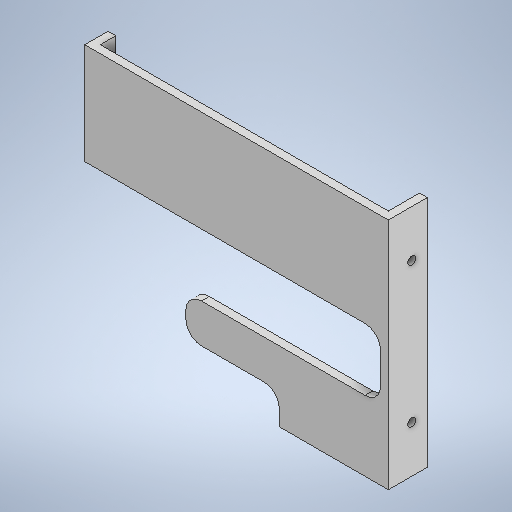
# Autodesk Inventor part: tright
Saved by Autodesk Inventor 2026.1 (Build 301233000, 233)
## iProperties
Created: 2026-05-31
Part Number: tright
Material: Generic
Document SubType Name: Modeling
Designer: chris
Density: 1 g/cm^3
Appearance: Default
Author: chris
Autodesk Inventor part; units mm, degrees
ref_plane "YZ Plane" through (0, 0, 0) normal (1, 0, 0) x (0, 1, 0)
ref_plane "XZ Plane" through (0, 0, 0) normal (0, 1, 0) x (-1, 0, 0)
ref_plane "XY Plane" through (0, 0, 0) normal (0, 0, 1) x (1, 0, 0)
sketch "Sketch1" plane through (0, 0, 0) normal (0, 0, 1) x (1, 0, 0)
  line L0 (-97.5, -75) -> (97.5, -75)
  line L1 (97.5, -75) -> (97.5, 75)
  line L2 (97.5, 75) -> (-97.5, 75)
  line L3 (-97.5, 75) -> (-97.5, -75)
  line L4 (-97.5, -75) -> (-32.5, -30) construction
  line L5 (97.5, -75) -> (-97.5, 75) construction
  line L6 (-97.5, -75) -> (-32.5, -75)
  line L7 (-32.5, -45) -> (-32.5, -40)
  line L8 (-42.5, 10) -> (-97.5, 10)
  line L9 (-97.5, 10) -> (-97.5, -75)
  line L10 (-97.5, -75) -> (27.5, -75)
  line L11 (27.5, -75) -> (27.5, -65)
  line L12 (17.5, -55) -> (-22.5, -55)
  line L13 (-97.5, -55) -> (-97.5, -75)
  arc A0 (-32.5, -45) -> (-22.5, -55) centre (-22.5, -45) ccw
  arc A1 (27.5, -65) -> (17.5, -55) centre (17.5, -65) ccw
  line L14 (-42.5, 10) -> (82.5, 10)
  line L15 (92.5, 0) -> (92.5, -20)
  line L16 (82.5, -30) -> (-22.5, -30)
  line L17 (-32.5, -30) -> (97.5, 75) construction
  arc A2 (-22.5, -30) -> (-32.5, -40) centre (-22.5, -40) ccw
  arc A3 (82.5, -30) -> (92.5, -20) centre (82.5, -20) ccw
  arc A4 (92.5, 0) -> (82.5, 10) centre (82.5, 0) ccw
  point P0 (0, 0)
  point P1 (-32.5, 10)
  point P2 (27.5, -55)
  point P3 (92.5, -30)
  point P4 (92.5, 10)
  dimension "d0" = 195
  dimension "d1" = 150
  dimension "d2" = 65
  dimension "d3" = 85
  dimension "d4" = 125
  dimension "d5" = 20
  dimension "d36" = 40
  dimension "d37" = 190
  dimension "d38" = 10
  constraints: 36 end point, 12 point on line, 10 point on circle, 10 tangent, 7 parallel, 5 centre point, 4 horizontal, 4 perpendicular, 3 equal radius, 1 midpoint
  measures "d0" distance of L2.end L1.end
  measures "d1" distance of L0.end L1.end
  measures "d2" distance of L8.end point (-32.5, 10)
  measures "d3" distance of point (-32.5, 10) L6.end
  measures "d4" distance of L13.start point (27.5, -55)
  measures "d5" distance of point (27.5, -55) L10.end
  measures "d36" distance of point (92.5, 10) point (92.5, -30)
  measures "d37" distance between parallel lines of L15 L9
  measures "d38" radius of A2
extrude "Extrusion1" add sketch "Sketch1" along normal blind 5 contours L11 A1 L12 A0 L7 A2 L16 A3 L15 A4 L14 L8 L3 L2 L1 L0
sketch "Sketch2" plane through (0, 0, 0) normal (0, 0, -1) x (-1, 0, 0)
  line L0 (92.5, 75) -> (97.5, 75)
  line L1 (97.5, 75) -> (97.5, 10)
  line L2 (97.5, 10) -> (92.5, 10)
  line L3 (92.5, 10) -> (92.5, 75)
  line L4 (-97.5, 75) -> (97.5, 75) projected
  line L5 (97.5, 10) -> (-82.5, 10) projected
  line L6 (97.5, 75) -> (97.5, 10) projected
  point P0 (0, 0)
  point P1 (42.5, 5)
  point P2 (97.5, -75)
  point P3 (-82.5, 10)
  dimension "d9" = 5
  constraints: 8 end point, 2 collinear, 2 horizontal, 2 parallel, 1 perpendicular, 1 other
  measures "d9" distance of L1.end L2.end
extrude "Extrusion2" add sketch "Sketch2" along normal blind 10
sketch "Sketch3" plane through (0, 0, 0) normal (0, 0, -1) x (-1, 0, 0)
  line L0 (-97.5, 75) -> (-92.5, 75)
  line L1 (-92.5, 75) -> (-92.5, -75)
  line L2 (-92.5, -75) -> (-97.5, -75)
  line L3 (-97.5, -75) -> (-97.5, 75)
  line L4 (-97.5, -70) -> (-27.5, -70)
  line L5 (-27.5, -70) -> (-27.5, -75)
  line L6 (-27.5, -75) -> (-97.5, -75)
  line L7 (-97.5, -75) -> (-97.5, -70)
  line L8 (-97.5, -75) -> (-97.5, 75) projected
  line L9 (-97.5, 75) -> (92.5, 75) projected
  line L10 (-27.5, -75) -> (-97.5, -75) projected
  line L11 (-27.5, -65) -> (-27.5, -75) projected
  point P0 (0, 0)
  point P1 (-92.5, -70)
  point P2 (97.5, -75)
  dimension "d12" = 5
  dimension "d13" = 5
  constraints: 16 end point, 5 collinear, 4 parallel, 2 horizontal, 2 perpendicular, 1 point on line
  measures "d12" distance of L0.start L0.end
  measures "d13" distance of L4.end L5.end
extrude "Extrusion3" add sketch "Sketch3" along normal blind 20
sketch "Sketch4" plane through (97.5, -75, 5) normal (1, 0, 0) x (0, 0, -1)
  circle A0 centre (15, 30) radius 2.55
  circle A1 centre (15, 120) radius 2.55
  line L0 (0, 0) -> (0, 150) projected
  line L1 (25, 0) -> (0, 0) projected
  point P0 (5, 75)
  dimension "d16" = 5.1
  dimension "d17" = 5.1
  dimension "d18" = 15
  dimension "d19" = 30
  dimension "d20" = 90
  constraints: 2 centre point, 1 vertical alignment
  measures "d16" diameter of A0
  measures "d17" diameter of A1
  measures "d18" distance from line of L0 A0.centre
  measures "d19" distance from line of L1 A0.centre
  measures "d20" distance of A0.centre A1.centre
extrude "Extrusion4" cut sketch "Sketch4" against normal blind 20
sketch "Sketch5" plane through (27.5, -75, 5) normal (0, -1, 0) x (1, 0, 0)
  circle A0 centre (35, -15) radius 2.55
  line L0 (70, -25) -> (70, 0) projected
  line L1 (0, 0) -> (70, 0) projected
  point P0 (-27.5, -5)
  point P1 (70, -12.5)
  point P2 (35, 0)
  point P3 (-125, 0)
  dimension "d23" = 5.1
  dimension "d24" = 35
  dimension "d25" = 15
  constraints: 2 midpoint, 1 centre point
  measures "d23" diameter of A0
  measures "d24" horizontal distance of point (70, -12.5) A0.centre
  measures "d25" distance of point (35, 0) A0.centre
extrude "Extrusion5" cut sketch "Sketch5" against normal blind 20
sketch "Sketch6" plane through (-97.5, 10, 5) normal (-1, 0, 0) x (0, 0, 1)
  circle A0 centre (-10, 45) radius 2.05
  circle A1 centre (-10, 20) radius 2.05
  line L0 (-15, 0) -> (-15, 65) projected
  line L1 (-15, 0) -> (0, 0) projected
  line L2 (0, 65) -> (-15, 65) projected
  point P0 (-5, -10)
  dimension "d28" = 4.1
  dimension "d29" = 4.1
  dimension "d30" = 5
  dimension "d31" = 20
  dimension "d32" = 20
  constraints: 2 centre point, 1 vertical alignment
  measures "d28" diameter of A0
  measures "d29" diameter of A1
  measures "d30" distance from line of L0 A1.centre
  measures "d31" distance from line of L1 A1.centre
  measures "d32" distance from line of L2 A0.centre
extrude "Extrusion6" cut sketch "Sketch6" against normal blind 20
body "Solid1"
